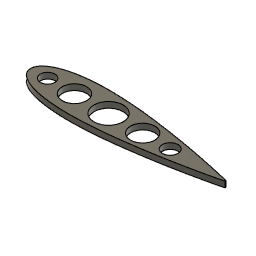
rib_nospar (Autodesk Fusion 360 design; units mm, degrees)
Autodesk Fusion 360 part; units mm, degrees
sketch "Sketch1" plane through (0, 0, 0) normal (0, 1, 0) x (1, 0, 0)
  circle A0 centre (45, 0) radius 12.5
  circle A1 centre (143.2403, 0) radius 8
  circle A2 centre (115, 0) radius 12.5
  circle A3 centre (17.5, 0) radius 7.5
  spline S0 degree 5 poles (200, 0.442) (199.5349, 0.5546) (198.6142, 0.7771) (197.2617, 1.103) (195.5156, 1.5218) (193.4243, 2.0198) (191.4115, 2.495) (189.4526, 2.9528) (187.5051, 3.4019) (185.509, 3.8552) (183.3993, 4.3263) (181.1175, 4.8274) (178.6226, 5.3668) (175.9043, 5.946) (172.9837, 6.5597) (169.9021, 7.1983) (166.7141, 7.8492) (163.4783, 8.4993) (160.249, 9.1365) (157.0682, 9.7517) (153.9563, 10.3407) (150.9161, 10.9035) (147.9371, 11.4428) (145.0001, 11.9633) (142.0821, 12.4703) (139.1599, 12.9686) (136.2156, 13.4615) (133.2392, 13.95) (130.2271, 14.4333) (127.1814, 14.9094) (124.1082, 15.3759) (121.0171, 15.83) (117.9195, 16.2692) (114.8283, 16.6922) (111.7556, 17.0983) (108.7119, 17.4875) (105.7037, 17.8601) (102.7328, 18.2165) (99.7938, 18.557) (96.8732, 18.8812) (93.9476, 19.1882) (90.9896, 19.4767) (87.9733, 19.7449) (84.8792, 19.9909) (81.7005, 20.213) (78.4473, 20.4095) (75.154, 20.5792) (71.8773, 20.7215) (68.6831, 20.836) (65.6373, 20.9226) (62.7944, 20.9816) (60.1868, 21.0131) (57.815, 21.0176) (55.6351, 20.9954) (53.5753, 20.9468) (51.5571, 20.8725) (49.5124, 20.7736) (47.4055, 20.652) (45.2448, 20.5097) (43.061, 20.3486) (40.8911, 20.1683) (38.7615, 19.966) (36.6665, 19.7341) (34.5722, 19.4623) (32.439, 19.1408) (30.239, 18.7629) (27.9748, 18.3286) (25.7002, 17.8477) (23.4982, 17.3363) (21.4536, 16.8128) (19.6289, 16.2935) (18.0357, 15.7888) (16.6175, 15.2995) (15.2858, 14.8132) (13.9485, 14.303) (12.5439, 13.7217) (11.0505, 13.0221) (9.4884, 12.1818) (7.9289, 11.2337) (6.4838, 10.2684) (5.2468, 9.368) (4.2539, 8.5628) (3.414, 7.7584) (2.5815, 6.7898) (1.6751, 5.516) (0.7924, 3.9084) (0.1283, 2.0295) (-0.1251, 0) (0.1283, -2.0295) (0.7924, -3.9084) (1.6751, -5.516) (2.5815, -6.7898) (3.414, -7.7584) (4.2539, -8.5628) (5.2468, -9.368) (6.4838, -10.2684) (7.9289, -11.2337) (9.4884, -12.1818) (11.0505, -13.0221) (12.5439, -13.7217) (13.9485, -14.303) (15.2858, -14.8132) (16.6175, -15.2995) (18.0357, -15.7888) (19.6289, -16.2935) (21.4536, -16.8128) (23.4982, -17.3363) (25.7002, -17.8477) (27.9748, -18.3286) (30.239, -18.7629) (32.439, -19.1408) (34.5722, -19.4623) (36.6665, -19.7341) (38.7615, -19.966) (40.8911, -20.1683) (43.061, -20.3486) (45.2448, -20.5097) (47.4055, -20.652) (49.5124, -20.7736) (51.5571, -20.8725) (53.5753, -20.9468) (55.6351, -20.9954) (57.815, -21.0176) (60.1868, -21.0131) (62.7944, -20.9816) (65.6373, -20.9226) (68.6831, -20.836) (71.8773, -20.7215) (75.154, -20.5792) (78.4473, -20.4095) (81.7005, -20.213) (84.8792, -19.9909) (87.9733, -19.7449) (90.9896, -19.4767) (93.9476, -19.1882) (96.8732, -18.8812) (99.7938, -18.557) (102.7328, -18.2165) (105.7037, -17.8601) (108.7119, -17.4875) (111.7556, -17.0983) (114.8283, -16.6922) (117.9195, -16.2692) (121.0171, -15.83) (124.1082, -15.3759) (127.1814, -14.9094) (130.2271, -14.4333) (133.2392, -13.95) (136.2156, -13.4615) (139.1599, -12.9686) (142.0821, -12.4703) (145.0001, -11.9633) (147.9371, -11.4428) (150.9161, -10.9035) (153.9563, -10.3407) (157.0682, -9.7517) (160.249, -9.1365) (163.4783, -8.4993) (166.7141, -7.8492) (169.9021, -7.1983) (172.9837, -6.5597) (175.9043, -5.946) (178.6226, -5.3668) (181.1175, -4.8274) (183.3993, -4.3263) (185.509, -3.8552) (187.5051, -3.4019) (189.4526, -2.9528) (191.4115, -2.495) (193.4243, -2.0198) (195.5156, -1.5218) (197.2617, -1.103) (198.6142, -0.7771) (199.5349, -0.5546) (200, -0.442) knots 0 0 0 0 0 0 0.00588235 0.01176471 0.01764706 0.02352941 0.02941176 0.03529412 0.04117647 0.04705882 0.05294118 0.05882353 0.06470588 0.07058824 0.07647059 0.08235294 0.08823529 0.09411765 0.1 0.10588235 0.11176471 0.11764706 0.12352941 0.12941176 0.13529412 0.14117647 0.14705882 0.15294118 0.15882353 0.16470588 0.17058824 0.17647059 0.18235294 0.18823529 0.19411765 0.2 0.20588235 0.21176471 0.21764706 0.22352941 0.22941176 0.23529412 0.24117647 0.24705882 0.25294118 0.25882353 0.26470588 0.27058824 0.27647059 0.28235294 0.28823529 0.29411765 0.3 0.30588235 0.31176471 0.31764706 0.32352941 0.32941176 0.33529412 0.34117647 0.34705882 0.35294118 0.35882353 0.36470588 0.37058824 0.37647059 0.38235294 0.38823529 0.39411765 0.4 0.40588235 0.41176471 0.41764706 0.42352941 0.42941176 0.43529412 0.44117647 0.44705882 0.45294118 0.45882353 0.46470588 0.47058824 0.47647059 0.48235294 0.48823529 0.49411765 0.5 0.50588235 0.51176471 0.51764706 0.52352941 0.52941176 0.53529412 0.54117647 0.54705882 0.55294118 0.55882353 0.56470588 0.57058824 0.57647059 0.58235294 0.58823529 0.59411765 0.6 0.60588235 0.61176471 0.61764706 0.62352941 0.62941176 0.63529412 0.64117647 0.64705882 0.65294118 0.65882353 0.66470588 0.67058824 0.67647059 0.68235294 0.68823529 0.69411765 0.7 0.70588235 0.71176471 0.71764706 0.72352941 0.72941176 0.73529412 0.74117647 0.74705882 0.75294118 0.75882353 0.76470588 0.77058824 0.77647059 0.78235294 0.78823529 0.79411765 0.8 0.80588235 0.81176471 0.81764706 0.82352941 0.82941176 0.83529412 0.84117647 0.84705882 0.85294118 0.85882353 0.86470588 0.87058824 0.87647059 0.88235294 0.88823529 0.89411765 0.9 0.90588235 0.91176471 0.91764706 0.92352941 0.92941176 0.93529412 0.94117647 0.94705882 0.95294118 0.95882353 0.96470588 0.97058824 0.97647059 0.98235294 0.98823529 0.99411765 1 1 1 1 1 1
  line L0 (0, 0) -> (200, 0) construction
  line L1 (200, 0.442) -> (200, -0.442)
  circle A4 centre (80, 0) radius 15
  spline S1 degree 3 poles (193.2694, 0) (192.485, 0.1862) (191.7212, 0.3667) (190.9675, 0.5437) (187.5367, 1.3495) (184.379, 2.0707) (180.1881, 2.9808) (177.3354, 3.6003) (173.9874, 4.3105) (170.3475, 5.0621) (166.284, 5.9012) (161.9294, 6.7754) (157.7781, 7.5756) (153.2067, 8.4567) (148.884, 9.2485) (144.6551, 9.9907) (140.0569, 10.7978) (135.4847, 11.567) (130.7466, 12.3225) (123.1082, 13.5405) (115.1003, 14.6738) (107.4756, 15.6237) (102.817, 16.204) (98.337, 16.7281) (93.7983, 17.1876) (89.7706, 17.5955) (85.6204, 17.9502) (81.2158, 18.2326) (76.913, 18.5083) (72.3744, 18.714) (68.237, 18.8434) (65.0227, 18.9439) (62.0959, 18.999) (59.5805, 19.0102) (56.5494, 19.0238) (54.0888, 18.9735) (51.5563, 18.8648) (49.3556, 18.7703) (47.0514, 18.6321) (44.6931, 18.4611) (42.3034, 18.2878) (39.9346, 18.0856) (37.648, 17.8254) (35.2743, 17.5552) (32.9116, 17.2095) (30.3864, 16.7455) (27.9401, 16.2961) (25.361, 15.738) (23.1353, 15.1722) (21.3364, 14.7149) (19.8145, 14.2625) (18.5154, 13.8303) (16.9821, 13.3201) (15.6691, 12.8402) (14.2545, 12.2578) (13.0842, 11.7759) (11.8388, 11.1916) (10.5506, 10.4582) (9.0995, 9.6321) (7.6417, 8.6527) (6.6017, 7.8631) (5.7975, 7.2525) (5.2613, 6.7824) (4.7168, 6.1772) (4.2242, 5.6298) (3.6737, 4.9138) (3.1638, 4.0085) (2.5517, 2.9219) (2.0707, 1.607) (2.0079, 0.3215) (1.948, -0.9036) (2.2649, -2.1627) (2.7893, -3.2825) (3.2592, -4.2861) (3.8509, -5.1377) (4.3708, -5.7736) (4.9864, -6.5265) (5.514, -7.0157) (6.3423, -7.6633) (7.2899, -8.4042) (8.645, -9.3362) (10.0527, -10.1692) (11.3728, -10.9503) (12.6799, -11.5932) (13.8923, -12.1065) (15.3747, -12.7343) (16.7331, -13.2305) (18.3014, -13.7586) (19.5822, -14.1899) (21.068, -14.6394) (22.842, -15.0971) (25.3044, -15.7324) (28.2319, -16.3625) (30.9585, -16.8491) (34.0519, -17.4013) (36.8894, -17.7702) (39.8682, -18.0583) (42.4461, -18.3076) (45.1563, -18.507) (47.746, -18.6648) (49.9639, -18.7998) (52.0409, -18.8996) (54.177, -18.9563) (56.3729, -19.0145) (58.7073, -19.028) (61.5054, -18.994) (64.7363, -18.9547) (68.58, -18.8517) (72.6137, -18.6838) (76.4943, -18.5223) (80.4767, -18.3003) (84.2332, -18.0256) (90.1037, -17.5964) (95.4623, -17.0423) (100.9626, -16.4065) (106.1231, -15.81) (111.4639, -15.1386) (116.8877, -14.3894) (122.4255, -13.6244) (127.9837, -12.7764) (133.3425, -11.9042) (138.3858, -11.0834) (143.2309, -10.2553) (148.2397, -9.3536) (151.9402, -8.6874) (155.7796, -7.9682) (159.7696, -7.1892) (164.0482, -6.3539) (168.4807, -5.4537) (172.4918, -4.6171) (175.7497, -3.9376) (178.69, -3.3092) (181.2285, -2.7541) (184.6524, -2.0054) (187.3934, -1.3802) (190.2821, -0.7044) (191.2574, -0.4762) (192.2462, -0.2429) (193.2694, 0) knots 0.01682571 0.01682571 0.01682571 0.01682571 0.0235295 0.0235295 0.0235295 0.05404421 0.05404421 0.05404421 0.07481524 0.07481524 0.07481524 0.09800339 0.09800339 0.09800339 0.12353747 0.12353747 0.12353747 0.15130166 0.15130166 0.15130166 0.19606145 0.19606145 0.19606145 0.22340899 0.22340899 0.22340899 0.24767746 0.24767746 0.24767746 0.27138504 0.27138504 0.27138504 0.28980289 0.28980289 0.28980289 0.31199655 0.31199655 0.31199655 0.33128188 0.33128188 0.33128188 0.35082424 0.35082424 0.35082424 0.37111098 0.37111098 0.37111098 0.39076376 0.39076376 0.39076376 0.40664722 0.40664722 0.40664722 0.42539433 0.42539433 0.42539433 0.44090494 0.44090494 0.44090494 0.45837666 0.45837666 0.45837666 0.47188613 0.47188613 0.47188613 0.48410685 0.48410685 0.48410685 0.49877673 0.49877673 0.49877673 0.51275909 0.51275909 0.51275909 0.52528941 0.52528941 0.52528941 0.54012411 0.54012411 0.54012411 0.5570968 0.5570968 0.5570968 0.5730128 0.5730128 0.5730128 0.5924742 0.5924742 0.5924742 0.60836694 0.60836694 0.60836694 0.63042624 0.63042624 0.63042624 0.65545321 0.65545321 0.65545321 0.67711193 0.67711193 0.67711193 0.69566076 0.69566076 0.69566076 0.71472769 0.71472769 0.71472769 0.73674491 0.73674491 0.73674491 0.75792665 0.75792665 0.75792665 0.79102815 0.79102815 0.79102815 0.82208435 0.82208435 0.82208435 0.85379338 0.85379338 0.85379338 0.88363575 0.88363575 0.88363575 0.90568383 0.90568383 0.90568383 0.92932655 0.92932655 0.92932655 0.94852947 0.94852947 0.94852947 0.97442994 0.97442994 0.97442994 0.98317429 0.98317429 0.98317429 0.98317429
  point P0 (160, -9.182)
  point P1 (140, -12.824)
  point P2 (190, -2.824)
  point P3 (180, -5.068)
  point P4 (15, 14.7)
  point P5 (10, -12.442)
  point P6 (2.5, 6.63)
  point P7 (5, 9.152)
  point P8 (10, 12.442)
  point P9 (100, -18.53)
  point P10 (5, -9.152)
  point P11 (2.5, -6.63)
  point P12 (50, 20.794)
  point P13 (30, 18.708)
  point P14 (20, 16.39)
  point P15 (40, 20.08)
  point P16 (60, -21.008)
  point P17 (80, -20.312)
  point P18 (180, 5.068)
  point P19 (190, 2.824)
  point P20 (20, -16.39)
  point P21 (30, -18.708)
  point P22 (40, -20.08)
  point P23 (50, -20.794)
  point P24 (120, 15.972)
  point P25 (100, 18.53)
  point P26 (80, 20.312)
  point P27 (60, 21.008)
  point P28 (140, 12.824)
  point P29 (160, 9.182)
  point P30 (15, -14.7)
  point P31 (120, -15.972)
  dimension "d14" = 25
  dimension "d15" = 16
  dimension "d16" = 25
  dimension "d17" = 30
  dimension "d19" = -2
  constraint coincident L0.start origin
  constraint horizontal L0
  constraint perpendicular L0 L1
  constraint coincident A0.centre L0
  constraint coincident A1.centre L0
  constraint coincident A2.centre L0
  constraint coincident A4.centre L0
  measures "d14" diameter of A0
  measures "d15" diameter of A1
  measures "d16" diameter of A2
  measures "d17" diameter of A4
extrude "Extrude2" add sketch "Sketch1" along normal blind 6 contours S0 L1 | S1
